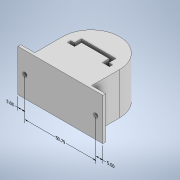
# Autodesk Inventor part: Part_B7
Saved by Autodesk Inventor 2022.6 (Build 266554010, 554A)
## iProperties
Created: 2025-05-30
Part Number: Part_B7
Material: Generic
Document SubType Name: Modeling
Designer: khinm
Density: 1 g/cm^3
Appearance: Default
Author: khinm
Autodesk Inventor part; units mm, degrees
ref_plane "YZ Plane" through (0, 0, 0) normal (1, 0, 0) x (0, 1, 0)
ref_plane "XZ Plane" through (0, 0, 0) normal (0, 1, 0) x (-1, 0, 0)
ref_plane "XY Plane" through (0, 0, 0) normal (0, 0, 1) x (1, 0, 0)
sketch "Sketch1" plane through (0, 0, 0) normal (0, 1, 0) x (-1, 0, 0)
  line L0 (-20.3963, -7) -> (-20.3963, 13)
  line L1 (-20.3963, 15) -> (20.3963, 15)
  line L2 (20.3963, 13) -> (20.3963, -7)
  arc A0 (-20.3963, -7) -> (20.3963, -7) centre (0, -7) ccw
  line L3 (20.3963, 15) -> (30.3963, 15)
  line L4 (30.3963, 15) -> (30.3963, 13)
  line L5 (30.3963, 13) -> (20.3963, 13)
  line L6 (-20.3963, 15) -> (-30.3963, 15)
  line L7 (-30.3963, 15) -> (-30.3963, 13)
  line L8 (-30.3963, 13) -> (-20.3963, 13)
  point P0 (0, 0)
  point P1 (0, 15)
  point P2 (20.3963, 0)
  dimension "d1" = 2
  dimension "d2" = 2
  dimension "d3" = 10
  dimension "d4" = 10
  dimension "d5" = 20
  dimension "d6" = 20.3963
  constraints: 18 end point, 3 parallel, 2 horizontal, 2 perpendicular, 2 point on circle, 2 vertical alignment, 1 centre point, 1 horizontal alignment, 1 midpoint, 1 point on line
  measures "d1" distance between parallel lines of L5 L3
  measures "d2" distance between parallel lines of L8 L6
  measures "d3" distance of L1.end L3.end
  measures "d4" distance of L1.start L6.end
  measures "d5" distance of L0.start L0.end
  measures "d6" radius of A0
extrude "Extrusion1" add sketch "Sketch1" along normal mid plane 30
sketch "Sketch2" plane through (0, 15, 0) normal (0, 1, 0) x (1, 0, 0)
  line L0 (-15, 5.0963) -> (-10, 5.0963)
  line L1 (-10, 5.0963) -> (-10, 10.0963)
  line L2 (-10, 10.0963) -> (10, 10.0963)
  line L3 (10, 10.0963) -> (10, 5.0963)
  line L4 (10, 5.0963) -> (15, 5.0963)
  line L5 (15, 5.0963) -> (15, 7.3963)
  line L6 (15, 7.3963) -> (12.3, 7.3963)
  line L7 (12.3, 7.3963) -> (12.3, 12.3963)
  line L8 (12.3, 12.3963) -> (-12.3, 12.3963)
  line L9 (-12.3, 12.3963) -> (-12.3, 7.3963)
  line L10 (-12.3, 7.3963) -> (-15, 7.3963)
  line L11 (-15, 7.3963) -> (-15, 5.0963)
  arc A0 (20.3963, 7) -> (-20.3963, 7) centre (0, 7) ccw projected
  point P0 (0, 0)
  point P1 (0, 12.3963)
  point P2 (0, 10.0963)
  point P3 (0, 27.3963)
  point P4 (15, 6.2463)
  point P5 (-15, 6.2463)
  point P6 (10, 7.5963)
  point P7 (-10, 7.5963)
  point P8 (-12.5, 5.0963)
  point P9 (-13.65, 7.3963)
  dimension "d9" = 15
  dimension "d11" = 2.3
  dimension "d13" = 24.6
  dimension "d14" = 20
  dimension "d15" = 5
  dimension "d17" = 5
  dimension "d27" = 2.3
  constraints: 24 end point, 10 perpendicular, 8 midpoint, 2 equal length, 2 point on line, 2 vertical alignment, 1 horizontal, 1 point on circle
  measures "d9" distance of point (0, 27.396) point (0, 12.396)
  measures "d11" distance between parallel lines of L2 L8
  measures "d13" distance of L7.end L8.end
  measures "d14" distance of point (10, 7.596) point (-10, 7.596)
  measures "d15" distance of L8.end L9.end
  measures "d17" distance from line of L1 point (-15, 6.246)
  measures "d27" vertical distance of point (-12.5, 5.096) point (-13.65, 7.396)
extrude "Extrusion2" cut sketch "Sketch2" against normal blind 25
sketch "Sketch3" plane through (30.3963, 15, 13) normal (0, 0, -1) x (-1, 0, 0)
  line L0 (0, -30) -> (0, 0) projected
  line L1 (0, 0) -> (10, 0) projected
  point P0 (30.3963, -15)
  point P1 (5, -15)
  point P2 (0, -15)
  point P3 (5, 0)
  constraints: 2 midpoint, 1 horizontal alignment, 1 vertical alignment
hole "Hole1" at (25.3963, 0, 13) direction (0, 0, 1) diameter 3 depth 2
mirror "Mirror1" about plane through (0, 0, 0) normal (1, 0, 0) of "Hole1"
body "Solid1"
